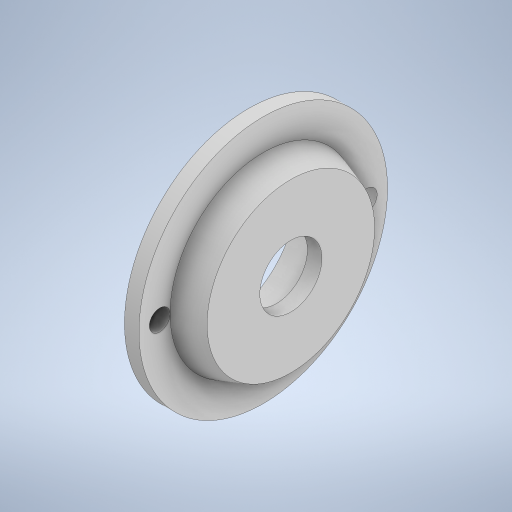
# Autodesk Inventor part: Cover
Saved by Autodesk Inventor 2024.3 (Build 283343000, 343)
## iProperties
Created: 2025-05-25
Part Number: Cover
Material: Generic
Document SubType Name: Modeling
Designer: Moaz
Density: 1 g/cm^3
Appearance: Default
Author: Moaz
Autodesk Inventor part; units mm, degrees
ref_plane "YZ Plane" through (0, 0, 0) normal (1, 0, 0) x (0, 1, 0)
ref_plane "XZ Plane" through (0, 0, 0) normal (0, 1, 0) x (-1, 0, 0)
ref_plane "XY Plane" through (0, 0, 0) normal (0, 0, 1) x (1, 0, 0)
sketch "Sketch1" plane through (0, 0, 0) normal (0, 0, 1) x (1, 0, 0)
  line L0 (-56.5702, 22.5) -> (-56.5702, 60.6429)
  line L1 (-56.5702, 60.6429) -> (-76.5702, 67.5)
  line L2 (-76.5702, 67.5) -> (-76.5702, 90)
  line L3 (-76.5702, 90) -> (-87.0702, 90)
  line L4 (-87.0702, 90) -> (-87.0702, 60)
  line L5 (-87.0702, 60) -> (-67.0702, 53.1429)
  line L6 (-67.0702, 53.1429) -> (-67.0702, 22.5)
  line L7 (-67.0702, 22.5) -> (-56.5702, 22.5)
  line L8 (-104.4843, 0) -> (17.414, 0) projected
  point P0 (0, 0)
  dimension "d11" = 22.5
  dimension "d12" = 90
  dimension "d13" = 60
  dimension "d17" = 20
  dimension "d18" = 56.5702
  dimension "d24" = 22.5
  dimension "d31" = 10.5
  dimension "d32" = 10.5
  dimension "d33" = 10.5
  constraints: 16 end point, 3 parallel, 3 perpendicular, 1 vertical
  measures "d11" distance between parallel lines of L7 L8
  measures "d12" distance between parallel lines of L3 L8
  measures "d13" distance from line of L8 L4.end
  measures "d17" distance between parallel lines of L6 L4
  measures "d18" distance from line of point (0, 0) L0
  measures "d24" distance of L1.end L2.end
  measures "d31" distance of L2.end L3.end
  measures "d32" distance of L6.end L0.start
  measures "d33" distance between parallel lines of L1 L5
revolve "Revolution1" add sketch "Sketch1" angle 360 about axis through (-10, 0, 0) along (1, 0, 0)
sketch "Sketch2" plane through (-76.5702, 0, 0) normal (1, 0, 0) x (0, 0, -1)
  circle A0 centre (0, 0) radius 67.5 projected
  circle A1 centre (0, 0) radius 75 construction
  circle A2 centre (-75, 0) radius 7.5
  circle A3 centre (75, 0) radius 7.5
  dimension "d21" = 150
  dimension "d22" = 15
  dimension "d23" = 15
  constraints: 3 centre point, 2 point on circle, 1 coincident
  measures "d21" diameter of A1
  measures "d22" diameter of A2
  measures "d23" diameter of A3
extrude "Extrusion1" cut sketch "Sketch2" against normal through all contours A2 | A3
sketch "Sketch3" plane through (-87.0702, 0, 0) normal (-1, 0, 0) x (0, 0, 1)
  circle A0 centre (0, 0) radius 60.6429 projected
  circle A1 centre (0, 0) radius 60
  circle A2 centre (0, 0) radius 55
  dimension "d27" = 120
  dimension "d28" = 110
  constraints: 2 centre point, 2 coincident
  measures "d27" diameter of A1
  measures "d28" diameter of A2
extrude "Extrusion2" add sketch "Sketch3" along normal mid plane 20 contours A1
sketch "Sketch4" plane through (-97.0702, 0, 0) normal (-1, 0, 0) x (0, 0, 1)
  circle A0 centre (0, 0) radius 55
  circle A1 centre (0, 0) radius 60
  dimension "d34" = 110
  dimension "d35" = 120
  constraints: 2 centre point, 2 coincident
  measures "d34" diameter of A0
  measures "d35" diameter of A1
extrude "Extrusion3" add sketch "Sketch4" along normal blind 10
body "Solid1"
